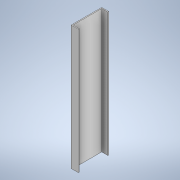
# Autodesk Inventor part: Tapa cable canal 150mm
Saved by Autodesk Inventor 2020 (Build 240168000, 168)
## iProperties
Created: 2020-10-14
Part Number: Tapa cable canal 150mm
Material: Genérico
Document SubType Name: Modeling
Designer: Pipi
Density: 1 g/cm^3
Appearance: Valor por defecto
Author: Pipi
Autodesk Inventor part; units mm, degrees
ref_plane "YZ Plane" through (0, 0, 0) normal (1, 0, 0) x (0, 1, 0)
ref_plane "XZ Plane" through (0, 0, 0) normal (0, 1, 0) x (-1, 0, 0)
ref_plane "XY Plane" through (0, 0, 0) normal (0, 0, 1) x (1, 0, 0)
sketch "Boceto1" plane through (0, 0, 0) normal (0, 1, 0) x (-1, 0, 0)
  line L0 (-5.4361, 12.1513) -> (1.0639, 12.1513)
  line L1 (1.0639, 12.1513) -> (1.0639, -17.8487)
  line L2 (1.0639, -17.8487) -> (-5.4361, -17.8487)
  line L3 (-5.4361, -17.8487) -> (-5.4361, -18.8487)
  line L4 (-5.4361, -18.8487) -> (2.0639, -18.8487)
  line L5 (2.0639, -18.8487) -> (2.0639, 13.1513)
  line L6 (2.0639, 13.1513) -> (-5.4361, 13.1513)
  line L7 (-5.4361, 13.1513) -> (-5.4361, 12.1513)
  point P0 (0, 0)
  point P1 (0, 0)
  dimension "d0" = 6.5
  dimension "d1" = 30
  dimension "d2" = 1
  dimension "d3" = 7.5
  dimension "d4" = 32
  constraints: 16 end point, 6 perpendicular, 1 horizontal, 1 parallel, 1 point on line
  measures "d0" distance of L0.start L0.end
  measures "d1" distance of L0.end L1.end
  measures "d2" distance of L2.end L3.end
  measures "d3" distance of L3.end L4.end
  measures "d4" distance of L4.end L5.end
extrude "Extrusión1" add sketch "Boceto1" along normal blind 130
